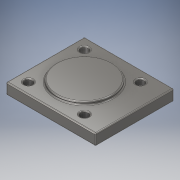
# Autodesk Inventor part: cylinderhead
Saved by Autodesk Inventor 2017 (Build 210142000, 142)
## iProperties
Created: 2020-01-04
Part Number: cylinderhead
Material: Stainless Steel
Document SubType Name: Modeling
Designer: Admin
Density: 8 g/cm^3
Appearance: Semi-Polished
Mass: 15.1426 g
Surface Area: 14.8034 cm^2
Volume: 1.89283 cm^3
Author: Admin
Autodesk Inventor part; units mm, degrees
ref_plane "YZ Plane" through (0, 0, 0) normal (1, 0, 0) x (0, 1, 0)
ref_plane "XZ Plane" through (0, 0, 0) normal (0, 1, 0) x (-1, 0, 0)
ref_plane "XY Plane" through (0, 0, 0) normal (0, 0, 1) x (1, 0, 0)
sketch "Sketch1" plane through (0, 0, 0) normal (0, 1, 0) x (-1, 0, 0)
  line L0 (-12.7, -11.1125) -> (12.7, -11.1125)
  line L1 (12.7, -11.1125) -> (12.7, 11.1125)
  line L2 (12.7, 11.1125) -> (-12.7, 11.1125)
  line L3 (-12.7, 11.1125) -> (-12.7, -11.1125)
  line L4 (12.7, -11.1125) -> (-12.7, 11.1125) construction
  circle A0 centre (1.5875, 0) radius 7.9375
  circle A1 centre (9.5275, 7.9375) radius 1.1303
  circle A2 centre (9.525, -7.9375) radius 1.1303
  circle A3 centre (-6.35, 7.9375) radius 1.1303
  circle A4 centre (-6.35, -7.9375) radius 1.1303
  point P0 (0, 0)
  dimension "d0" = 22.225
  dimension "d1" = 25.4
  dimension "d2" = 15.875
  dimension "d11" = 11.1125
  dimension "d12" = 2.2606
  dimension "d13" = 2.2606
  dimension "d14" = 2.2606
  dimension "d15" = 2.2606
  dimension "d16" = 15.875
  dimension "d17" = 15.8775
  dimension "d18" = 15.875
  dimension "d19" = 7.9375
  dimension "d20" = 7.9375
  dimension "d31" = 12.7
  dimension "d32" = 3.1725
  dimension "d33" = 3.175
  dimension "d34" = 3.175
  dimension "d35" = 19.05
  constraints: 10 end point, 5 centre point, 2 parallel, 1 horizontal, 1 midpoint, 1 perpendicular
  measures "d0" distance of L0.end L1.end
  measures "d1" distance of L0.start L0.end
  measures "d2" diameter of A0
  measures "d11" distance from line of L1 A0.centre
  measures "d12" diameter of A1
  measures "d13" diameter of A2
  measures "d14" diameter of A3
  measures "d15" diameter of A4
  measures "d16" distance of A2.centre A4.centre
  measures "d17" distance of A1.centre A3.centre
  measures "d18" distance of A4.centre A3.centre
  measures "d19" horizontal distance of A0.centre A4.centre
  measures "d20" horizontal distance of A0.centre A4.centre
  measures "d31" distance from line of point (0, 0) L1
  measures "d32" distance from line of A1.centre L1
  measures "d33" distance from line of A1.centre L2
  measures "d34" distance from line of A2.centre L1
  measures "d35" distance from line of A2.centre L2
extrude "Extrusion1" add sketch "Sketch1" along normal blind 3.175
extrude "Extrusion2" add sketch "Sketch1" along normal blind 3.9688 contours A0
fillet "Fillet1" radius 0.3175 22 edges at (7.4803, 3.175, -7.9375) (7.4803, 0, -7.9375) (7.4803, 3.175, 7.9375) (7.4803, 0, 7.9375) (-8.3947, 3.175, -7.9375) (-8.3947, 0, -7.9375) (-8.3972, 3.175, 7.9375) (-8.3972, 0, 7.9375) (12.7, 0, 0) (12.7, 1.5875, -11.1125) (12.7, 3.175, 0) (12.7, 1.5875, 11.1125) (0, 0, 11.1125) (0, 3.175, 11.1125) (-12.7, 1.5875, 11.1125) (-12.7, 0, 0) (-12.7, 3.175, 0) (-12.7, 1.5875, -11.1125) (0, 0, -11.1125) (0, 3.175, -11.1125) (6.35, 3.9688, 0) (6.35, 3.175, 0)
body "Solid1"
